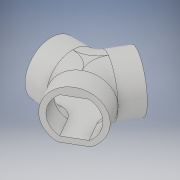
# Autodesk Inventor part: 3 way corridor
Saved by Autodesk Inventor 2017 (Build 210142000, 142)
## iProperties
Created: 2018-03-04
Part Number: 3 way corridor
Material: Generic
Document SubType Name: Modeling
Designer: Braxton
Density: 1 g/cm^3
Appearance: Default
Author: Braxton
Autodesk Inventor part; units mm, degrees
ref_plane "YZ Plane" through (0, 0, 0) normal (1, 0, 0) x (0, 1, 0)
ref_plane "XZ Plane" through (0, 0, 0) normal (0, 1, 0) x (-1, 0, 0)
ref_plane "XY Plane" through (0, 0, 0) normal (0, 0, 1) x (1, 0, 0)
sketch "Sketch1" plane through (0, 0, 0) normal (1, 0, 0) x (0, 1, 0)
  line L0 (84.666667, 50.8) -> (84.666667, -50.8)
  line L1 (-84.666667, 50.8) -> (-84.666667, -50.8)
  arc A0 (-110.066667, -57.405887) -> (-110.066667, 57.405887) centre (0, 0) ccw
  arc A1 (84.666667, 50.8) -> (-84.666667, 50.8) centre (0, 0) ccw
  arc A2 (-84.666667, -50.8) -> (84.666667, -50.8) centre (0, 0) ccw
  line L2 (-110.066667, 57.405887) -> (-110.066667, -57.405887)
  dimension "d10" = 169.33333
  dimension "d11" = 101.6
  dimension "d14" = 248.2749
  dimension "d46" = 25.4
  constraints: 6 end point, 6 point on circle, 3 centre point, 2 coincident, 1 parallel, 1 vertical
  measures "d10" distance between parallel lines of L1 L0
  measures "d11" distance of L0.start L0.end
  measures "d14" diameter of A0
  measures "d46" distance between parallel lines of L1 L2
extrude "corridor" add sketch "Sketch1" along normal blind 101.6
sketch "found rotaion axis" plane through (0, 0, 0) normal (0, 1, 0) x (-1, 0, 0)
  line L0 (-101.6, 124.137452) -> (-101.6, -124.137452)
  line L1 (-101.6, -124.137452) -> (-101.6, 124.137452)
  line L2 (-101.6, 0) -> (-173.270792, 0)
  point P0 (0, 0)
  dimension "d15" = 71.67079
  constraints: 4 end point, 1 horizontal, 1 midpoint, 1 vertical
  measures "d15" distance of L2.start L2.end
pattern_circular "other corridors" count 3 over 360 about axis through (173.270792, 0, 0) along (0, 1, 0) of "corridor"
sketch "Sketch4" plane through (0, 0, 0) normal (0, 1, 0) x (-1, 0, 0)
  line L0 (0, -98.737452) -> (-101.6, -98.737452)
  line L1 (-174.397046, -199.425634) -> (-123.597046, -111.437453)
  line L2 (-101.6, -98.737452) -> (0, -98.737452)
  line L3 (0, -124.137452) -> (0, 124.137452)
  line L4 (-123.597046, -111.437453) -> (-174.397046, -199.425634)
  line L5 (-367.412375, -87.988182) -> (-152.400001, -212.125634)
  line L6 (-345.41533, -100.688182) -> (-294.61533, -12.700001)
  line L7 (-345.41533, -100.688182) -> (-294.61533, -12.700001)
  line L8 (-345.41533, 100.688182) -> (-294.61533, 12.700001)
  line L9 (-294.615329, 12.7) -> (-312.526979, 43.723888)
  line L10 (-174.397046, 199.425634) -> (-123.597046, 111.437453)
  line L11 (-123.597046, 111.437453) -> (-165.112098, 87.468727)
  line L12 (-187.474467, 222.076391) -> (-123.597046, 111.437453)
  line L13 (0, 98.737452) -> (-101.6, 98.737452)
  line L14 (-101.600001, 98.737452) -> (0, 98.737452)
  line L15 (-101.600001, -124.137453) -> (-316.612375, -0.000001)
  arc A0 (-101.600001, -98.737452) -> (-123.597047, -111.437452) centre (-101.600001, -124.137453) ccw
  arc A1 (-294.61533, -12.700001) -> (-294.615329, 12.7) centre (-316.612375, -0.000001) ccw
  line L16 (-316.612376, 0) -> (-101.600001, 124.137453)
  arc A2 (-123.597046, 111.437453) -> (-101.600001, 98.737452) centre (-101.600001, 124.137453) ccw
  point P0 (0, 0)
  point P1 (-316.612375, -0.000001)
  point P2 (-244.941584, 103.912102)
  point P3 (-277.182894, 71.670792)
  constraints: 13 end point, 8 point on circle, 8 point on line, 3 centre point, 3 perpendicular, 1 coincident, 5 other
sketch "Sketch5" plane through (101.6, 0, 0) normal (1, 0, 0) x (0, 0, -1)
  arc A0 (50.8, -84.666667) -> (50.8, 84.666667) centre (0, 0) ccw
  arc A1 (0, -124.137452) -> (0, 124.137452) centre (0, 0) ccw
  line L0 (50.8, 84.666667) -> (0, 84.666667)
  line L1 (50.8, -84.666667) -> (0, -84.666667)
  line L2 (0, 124.137452) -> (0, 84.666667)
  line L3 (0, -84.666667) -> (0, -124.137452)
  constraints: 8 end point, 4 point on circle, 2 centre point, 2 coincident, 2 point on line, 2 vertical
sweep "curve edjes" add profiles "Sketch5" path "Sketch4" path curves A0
pattern_circular "repeat curve edjes" count 3 over 360 about axis through (173.270792, 0, 0) along (0, 1, 0) of "curve edjes"
sketch "Sketch7" plane through (0, -84.666667, 50.8) normal (0, 1, 0) x (1, 0, 0)
  arc A0 (209.106188, -11.268727) -> (101.6, 50.8) centre (101.6, -73.337452) ccw
  arc A1 (209.106188, -11.268727) -> (101.6, 50.8) centre (101.6, -73.337452) ccw
  arc A2 (101.6, 50.8) -> (209.106188, 112.868725) centre (101.600001, 174.937453) ccw
  line L0 (316.612375, 50.800001) -> (209.106188, -11.268727)
  arc A3 (209.106188, 112.868725) -> (209.106188, -11.268727) centre (316.612375, 50.799999) ccw
  arc A4 (209.106188, 112.868725) -> (209.106188, -11.268727) centre (316.612375, 50.799999) ccw
  line L1 (209.106188, 112.868725) -> (316.612375, 50.800001)
  arc A5 (101.6, 50.8) -> (209.106188, 112.868725) centre (101.600001, 174.937453) ccw
  point P0 (173.270792, 50.8)
  constraints: 6 point on circle, 3 centre point, 3 concentric
extrude "bottom hole fill up" add sketch "Sketch7" against normal blind 39.470785 contours A0 A2 A3
mirror "top hole fill up" about plane through (0, 0, 0) normal (0, 1, 0) of "bottom hole fill up"
body "Solid1"
